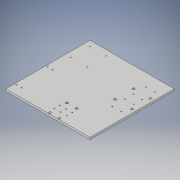
# Autodesk Inventor part: DPLX_P013_Lab_Baseplate
Saved by Autodesk Inventor 2018 (Build 220112000, 112)
## iProperties
Created: 2018-06-11
Part Number: DPLX_P013_Lab_Baseplate
Material: Generic
Document SubType Name: Modeling
Designer: DPLXuser
Density: 1 g/cm^3
Appearance: Default
Author: DPLXuser
Autodesk Inventor part; units mm, degrees
ref_plane "YZ Plane" through (0, 0, 0) normal (1, 0, 0) x (0, 1, 0)
ref_plane "XZ Plane" through (0, 0, 0) normal (0, 1, 0) x (-1, 0, 0)
ref_plane "XY Plane" through (0, 0, 0) normal (0, 0, 1) x (1, 0, 0)
sketch "Sketch1" plane through (0, 0, 0) normal (0, 1, 0) x (-1, 0, 0)
  line L0 (-127, 127) -> (127, 127)
  line L1 (127, 127) -> (127, -127)
  line L2 (127, -127) -> (-127, -127)
  line L3 (-127, -127) -> (-127, 127)
  line L4 (-127, 127) -> (127, -127) construction
  line L5 (127, 127) -> (-127, -127) construction
  point P0 (0, 0)
  dimension "d0" = 254
  dimension "d1" = 254
  constraints: 12 end point, 2 midpoint, 2 parallel, 1 horizontal, 1 perpendicular
  measures "d0" distance of L1.end L2.end
  measures "d1" distance of L0.end L1.end
extrude "Extrusion1" add sketch "Sketch1" along normal blind 6.35
sketch "Sketch4" plane through (0, 6.35, 0) normal (0, 1, 0) x (1, 0, 0)
  line L0 (127, -127) -> (127, 127) projected
  line L1 (127, 127) -> (-127, 127) projected
  circle A0 centre (80.01, -12.7) radius 1.4986
  circle A1 centre (80.01, 25.4) radius 1.4986
  circle A2 centre (80.01, 50.8) radius 1.4986
  circle A3 centre (80.01, 88.9) radius 1.4986
  circle A4 centre (106.68, -12.7) radius 1.4986
  circle A5 centre (106.68, 25.4) radius 1.4986
  circle A6 centre (106.68, 50.8) radius 1.4986
  circle A7 centre (106.68, 88.9) radius 1.4986
  point P0 (0, 0)
  dimension "d60" = 2.9972
  dimension "d61" = 2.9972
  dimension "d62" = 2.9972
  dimension "d63" = 2.9972
  dimension "d64" = 2.9972
  dimension "d65" = 2.9972
  dimension "d66" = 2.9972
  dimension "d67" = 2.9972
  constraints: 8 centre point
  measures "d60" diameter of A0
  measures "d61" diameter of A1
  measures "d62" diameter of A2
  measures "d63" diameter of A3
  measures "d64" diameter of A4
  measures "d65" diameter of A5
  measures "d66" diameter of A6
  measures "d67" diameter of A7
extrude "Extrusion4" cut sketch "Sketch4" against normal blind 6.35
sketch "Sketch5" plane through (0, 6.35, 0) normal (0, 1, 0) x (1, 0, 0)
  line L0 (127, 127) -> (127, -127) projected
  line L1 (127, 127) -> (116.7384, 127)
  line L2 (-127, 127) -> (127, 127) projected
  circle A0 centre (65.9384, 10.3124) radius 3.5052
  circle A1 centre (65.9384, 65.8622) radius 3.5052
  circle A2 centre (116.7384, 65.8622) radius 3.5052
  circle A3 centre (116.7384, 10.3124) radius 3.5052
  point P0 (0, 0)
  dimension "d70" = 10.2616
  dimension "d74" = 7.0104
  dimension "d75" = 7.0104
  dimension "d76" = 7.0104
  dimension "d77" = 7.0104
  constraints: 4 centre point, 2 end point, 1 point on line
  measures "d70" distance of L0.start L1.end
  measures "d74" diameter of A0
  measures "d75" diameter of A1
  measures "d76" diameter of A2
  measures "d77" diameter of A3
extrude "Extrusion5" cut sketch "Sketch5" against normal blind 6.35
sketch "Sketch6" plane through (0, 6.35, 0) normal (0, 1, 0) x (1, 0, 0)
  line L0 (127, 127) -> (127, -127) projected
  line L1 (127, -127) -> (-127, -127) projected
  circle A0 centre (2.159, -71.8312) radius 3.5052
  circle A1 centre (2.159, -122.6312) radius 3.5052
  circle A2 centre (31.369, -71.8312) radius 3.5052
  circle A3 centre (31.369, -122.6312) radius 3.5052
  point P0 (0, 0)
  dimension "d84" = 7.0104
  dimension "d85" = 7.0104
  dimension "d86" = 7.0104
  dimension "d87" = 7.0104
  constraints: 4 centre point
  measures "d84" diameter of A0
  measures "d85" diameter of A1
  measures "d86" diameter of A2
  measures "d87" diameter of A3
extrude "Extrusion6" cut sketch "Sketch6" against normal blind 6.35
sketch "Sketch7" plane through (0, 6.35, 0) normal (0, 1, 0) x (1, 0, 0)
  line L0 (127, 127) -> (127, -127) projected
  line L1 (-127, -127) -> (127, -127) projected
  circle A0 centre (16.764, -105.41) radius 1.4986
  circle A1 centre (-2.032, -105.41) radius 1.4986
  circle A2 centre (-2.032, -89.0524) radius 1.4986
  circle A3 centre (16.764, -89.0524) radius 1.4986
  circle A4 centre (35.56, -89.0524) radius 1.4986
  circle A5 centre (35.56, -105.41) radius 1.4986
  point P0 (0, 0)
  dimension "d95" = 2.9972
  dimension "d96" = 2.9972
  dimension "d97" = 2.9972
  dimension "d98" = 2.9972
  dimension "d99" = 2.9972
  dimension "d100" = 2.9972
  constraints: 6 centre point
  measures "d95" diameter of A0
  measures "d96" diameter of A1
  measures "d97" diameter of A2
  measures "d98" diameter of A3
  measures "d99" diameter of A4
  measures "d100" diameter of A5
extrude "Extrusion7" cut sketch "Sketch7" against normal blind 6.35
sketch "Sketch8" plane through (0, 6.35, 0) normal (0, 1, 0) x (1, 0, 0)
  line L0 (-127, 127) -> (-127, -127) projected
  circle A0 centre (-121.92, -6.477) radius 1.7018
  circle A1 centre (-121.92, -100.2792) radius 1.7018
  circle A2 centre (-105.9701, -100.2792) radius 1.7018
  circle A3 centre (-106.68, -6.477) radius 1.7018
  point P0 (0, 0)
  dimension "d108" = 3.4036
  dimension "d110" = 3.4036
  dimension "d124" = 3.4036
  dimension "d125" = 3.4036
  constraints: 4 centre point
  measures "d108" diameter of A0
  measures "d110" diameter of A1
  measures "d124" diameter of A2
  measures "d125" diameter of A3
extrude "Extrusion8" cut sketch "Sketch8" against normal blind 6.35
sketch "Sketch9" plane through (0, 6.35, 0) normal (0, 1, 0) x (1, 0, 0)
  line L0 (-127, 127) -> (-127, 110.7948)
  circle A0 centre (-110.7948, 110.7948) radius 1.3716
  circle A1 centre (-110.7948, 52.8066) radius 1.3716
  circle A2 centre (-61.7982, 52.8066) radius 1.3716
  circle A3 centre (-61.7982, 110.7948) radius 1.3716
  point P0 (0, 0)
  dimension "d113" = 16.2052
  dimension "d117" = 2.7432
  dimension "d118" = 2.7432
  dimension "d119" = 2.7432
  dimension "d120" = 2.7432
  constraints: 4 centre point, 2 end point
  measures "d113" distance of L0.start L0.end
  measures "d117" diameter of A0
  measures "d118" diameter of A1
  measures "d119" diameter of A2
  measures "d120" diameter of A3
extrude "Extrusion9" cut sketch "Sketch9" against normal blind 6.35
body "Solid1"
